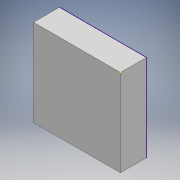
# Autodesk Inventor part: Bottom
Saved by Autodesk Inventor 2018 (Build 220112000, 112)
## iProperties
Created: 2018-04-10
Part Number: Bottom
Material: Generic
Document SubType Name: Modeling
Designer: a
Density: 1 g/cm^3
Appearance: Default
Author: a
Autodesk Inventor part; units mm, degrees
ref_plane "YZ Plane" through (0, 0, 0) normal (1, 0, 0) x (0, 1, 0)
ref_plane "XZ Plane" through (0, 0, 0) normal (0, 1, 0) x (-1, 0, 0)
ref_plane "XY Plane" through (0, 0, 0) normal (0, 0, 1) x (1, 0, 0)
sketch "Sketch1" plane through (0, 0, 0) normal (0, 1, 0) x (-1, 0, 0)
  point P0 (0, 0)
sketch "Sketch2" plane through (0, 0, 0) normal (0, 1, 0) x (-1, 0, 0)
  line L0 (0, 0) -> (150, 0)
  line L1 (150, 0) -> (150, -150)
  line L2 (150, -150) -> (0, -150)
  line L3 (0, -150) -> (0, 0)
  dimension "d0" = 150
  dimension "d1" = 150
  constraints: 8 end point, 2 parallel, 1 horizontal, 1 perpendicular
  measures "d0" distance of L1.end L2.end
  measures "d1" distance of L0.end L1.end
extrude "Extrusion1" add sketch "Sketch2" along normal blind 10
sketch "Sketch3" plane through (0, 10, 0) normal (0, 1, 0) x (1, 0, 0)
  line L0 (-150, 0) -> (0, 0) projected
  line L1 (0, 150) -> (-150, 150) projected
  line L2 (0, 0) -> (-150, 0)
  line L3 (-150, 0) -> (-150, 150)
  line L4 (-150, 150) -> (0, 150)
  line L5 (0, 150) -> (0, 0)
  line L6 (-145.7, 145.7) -> (-145.7, 4.3)
  line L7 (-145.7, 4.3) -> (-4.3, 4.3)
  line L8 (-4.3, 4.3) -> (-4.3, 145.7)
  line L9 (-4.3, 145.7) -> (-145.7, 145.7)
  dimension "d4" = 4.3
  constraints: 16 end point, 4 parallel, 2 perpendicular, 1 horizontal, 3 other
  measures "d4" distance between parallel lines of L3 L6
extrude "Extrusion2" add sketch "Sketch3" along normal blind 35
sketch "Sketch4" plane through (0, 45, 0) normal (0, 1, 0) x (1, 0, 0)
  line L0 (0, 0) -> (-150, 0) projected
  line L1 (-150, 150) -> (-150, 0) projected
  line L2 (0, 0) -> (-150, 0)
  line L3 (-150, 0) -> (-150, 150)
  line L4 (-150, 150) -> (0, 150)
  line L5 (0, 150) -> (0, 0)
  line L6 (-145.7, 4.3) -> (-145.7, 145.7) projected
  line L7 (-4.3, 4.3) -> (-145.7, 4.3) projected
  line L8 (-145.7, 145.7) -> (-4.3, 145.7)
  line L9 (-4.3, 145.7) -> (-4.3, 4.3)
  line L10 (-4.3, 4.3) -> (-145.7, 4.3)
  line L11 (-145.7, 4.3) -> (-145.7, 145.7)
  constraints: 16 end point, 4 parallel, 2 horizontal, 2 perpendicular
sketch "Sketch5" plane through (0, 0, 0) normal (1, 0, 0) x (0, 0, -1)
  point P0 (0, 0)
sketch "Sketch6" plane through (0, 0, 0) normal (1, 0, 0) x (0, 0, -1)
  point P0 (0, 0)
sketch "Sketch7" plane through (0, 0, 0) normal (1, 0, 0) x (0, 0, -1)
  point P0 (0, 0)
sketch "Sketch8" plane through (0, 0, 0) normal (1, 0, 0) x (0, 0, -1)
  point P0 (0, 0)
sketch "Sketch9" plane through (0, 0, 0) normal (1, 0, 0) x (0, 0, -1)
  point P0 (0, 0)
body "Solid1"
